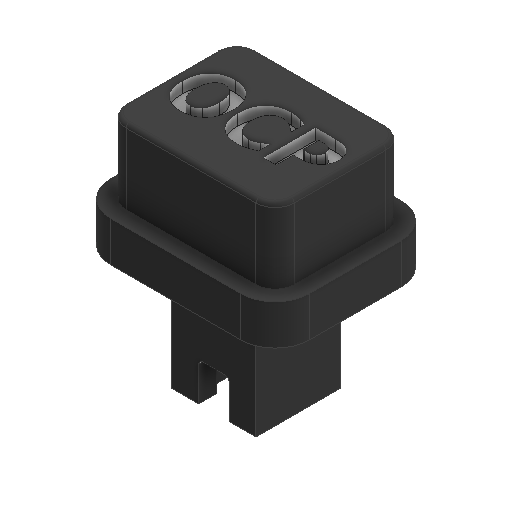
# Autodesk Inventor part: Button cap
Saved by Autodesk Inventor 2025 (Build 290162000, 162)
## iProperties
Created: 2025-01-02
Part Number: Button cap
Material: Generic
Document SubType Name: Modeling
Designer: Jan Mareš
Density: 1 g/cm^3
Appearance: Default
Author: Jan Mareš
Autodesk Inventor part; units mm, degrees
ref_plane "YZ Plane" through (0, 0, 0) normal (1, 0, 0) x (0, 1, 0)
ref_plane "XZ Plane" through (0, 0, 0) normal (0, 1, 0) x (-1, 0, 0)
ref_plane "XY Plane" through (0, 0, 0) normal (0, 0, 1) x (1, 0, 0)
sketch "Sketch1" plane through (0, 0, 0) normal (0, 1, 0) x (-1, 0, 0)
  line L0 (3.08, 0) -> (-3.08, 0) construction
  line L1 (0, -3.08) -> (0, 3.08) construction
  line L2 (-2.2, 2.2) -> (2.2, 2.2)
  line L3 (2.2, 2.2) -> (2.2, -2.2)
  line L4 (2.2, -2.2) -> (-2.2, -2.2)
  line L5 (-2.2, -2.2) -> (-2.2, 2.2)
  line L6 (-2.2, 0) -> (2.2, 0) construction
  point P0 (0, 0)
  dimension "d0" = 4.4
  constraints: 10 end point, 3 midpoint, 2 parallel, 2 perpendicular, 1 horizontal
  measures "d0" distance of L2.start L2.end
extrude "Extrusion1" add sketch "Sketch1" along normal blind 6
sketch "Sketch2" plane through (0, 0, 0) normal (0, -1, 0) x (1, 0, 0)
  line L0 (-1.25, 1.25) -> (1.25, 1.25)
  line L1 (1.25, 1.25) -> (1.25, -1.25)
  line L2 (1.25, -1.25) -> (-1.25, -1.25)
  line L3 (-1.25, -1.25) -> (-1.25, 1.25)
  line L4 (-1.25, 0) -> (1.25, 0) construction
  point P0 (0, 0)
  point P1 (0, 0)
  dimension "d3" = 2.5
  constraints: 10 end point, 3 midpoint, 2 parallel, 2 perpendicular, 1 coincident, 1 horizontal
  measures "d3" distance of L0.start L0.end
extrude "Extrusion2" cut sketch "Sketch2" against normal blind 2.8
sketch "Sketch3" plane through (-2.2, 0, 2.2) normal (0, 0, 1) x (1, 0, 0)
  line L0 (2.2, -1.2) -> (2.2, 7.2) construction
  line L1 (-0.88, 0) -> (5.28, 0) construction
  line L2 (1.4, 0) -> (1.4, 2)
  line L3 (1.4, 2) -> (3, 2)
  line L4 (3, 2) -> (3, 0)
  line L5 (1.4, 0) -> (3, 0)
  line L6 (1.4, 1) -> (3, 1) construction
  point P0 (2.2, 0)
  point P1 (2.2, 1)
  dimension "d6" = 1.6
  dimension "d7" = 2
  constraints: 10 end point, 3 midpoint, 3 point on line, 2 perpendicular, 1 collinear, 1 vertical
  measures "d6" distance of L2.end L3.end
  measures "d7" distance of L3.end L4.end
extrude "Extrusion3" cut sketch "Sketch3" against normal through all
sketch "Sketch4" plane through (0, 0, 0) normal (0, 0, 1) x (1, 0, 0)
  line L0 (1.25, 0) -> (1.25, 2.8) construction
  line L1 (-1.25, 0) -> (-1.25, 2.8) construction
  line L2 (-1.758, 0) -> (1.798, 0) construction
  arc A0 (1.25, 0.9) -> (1.25, 0.6317) centre (1.29, 0.7658) ccw
  line L3 (1.29, 0.7658) -> (1.15, 0.7658) construction
  line L4 (1.25, 0.6317) -> (1.25, 0.9) construction
  line L5 (1.1441, 0.9) -> (1.25, 0.9)
  line L6 (1.1441, 0.9) -> (1.25, 0.7165)
  line L7 (1.25, 0.9) -> (1.25, 0.7165)
  line L8 (1.25, 0.9) -> (1.25, 0.6317)
  point P0 (0, 0)
  dimension "d13" = 0.1
  dimension "d14" = 1.9
  dimension "d15" = 0.14
  dimension "d28" = 30
  dimension "d29" = 0.106
  dimension "d30" = 1.9
  constraints: 12 end point, 6 point on line, 3 point on circle, 1 centre point, 1 collinear, 1 horizontal, 1 perpendicular
  measures "d13" distance from line of L0 L3.end
  measures "d14" distance of L4.end L0.end
  measures "d15" radius of A0
  measures "d28" angle of L0 L6
  measures "d29" distance of L5.start L5.end
  measures "d30" distance from line of L5 L0.end
extrude "Extrusion4" add sketch "Sketch4" along normal through all both and the other way through all contours L7 L6 A0 | L6 L8 A0
mirror "Mirror1" about plane through (0, 0, 0) normal (1, 0, 0) of "Extrusion4"
sketch "Sketch5" plane through (0, 6, 0) normal (0, 1, 0) x (1, 0, 0)
  line L0 (-4.4, -3.4) -> (4.4, -3.4)
  line L1 (4.4, -3.4) -> (4.4, 3.4)
  line L2 (4.4, 3.4) -> (-4.4, 3.4)
  line L3 (-4.4, 3.4) -> (-4.4, -3.4)
  line L4 (0, -3.4) -> (0, 3.4) construction
  line L5 (6.16, 0) -> (-6.16, 0) construction
  point P0 (0, 0)
  dimension "d18" = 6.8
  dimension "d19" = 8.8
  constraints: 10 end point, 3 midpoint, 2 parallel, 1 horizontal, 1 perpendicular
  measures "d18" distance of L2.end L0.start
  measures "d19" distance of L0.start L0.end
extrude "Extrusion5" add sketch "Sketch5" along normal blind 6
fillet "Fillet1" radius 1 4 edges at (4.4, 9, 3.4) (4.4, 9, -3.4) (-4.4, 9, 3.4) (-4.4, 9, -3.4)
fillet "Fillet2" radius 0.2 8 edges at (4.1071, 12, -3.1071) (0, 12, -3.4) (-4.1071, 12, -3.1071) (-4.4, 12, 0) (-4.1071, 12, 3.1071) (0, 12, 3.4) (4.1071, 12, 3.1071) (4.4, 12, 0)
sketch "Sketch6" plane through (0, 6, 0) normal (0, -1, 0) x (1, 0, 0)
  line L0 (-3.4, 3.4) -> (3.4, 3.4) projected
  arc A0 (4.4, 2.4) -> (3.4, 3.4) centre (3.4, 2.4) ccw projected
  line L1 (4.4, 2.4) -> (4.4, -2.4) projected
  arc A1 (3.4, -3.4) -> (4.4, -2.4) centre (3.4, -2.4) ccw projected
  line L2 (3.4, -3.4) -> (-3.4, -3.4) projected
  arc A2 (-4.4, -2.4) -> (-3.4, -3.4) centre (-3.4, -2.4) ccw projected
  line L3 (-4.4, -2.4) -> (-4.4, 2.4) projected
  arc A3 (-3.4, 3.4) -> (-4.4, 2.4) centre (-3.4, 2.4) ccw projected
  line L4 (3.4, 4.2) -> (-3.4, 4.2)
  arc A4 (-3.4, 4.2) -> (-5.2, 2.4) centre (-3.4, 2.4) ccw
  line L5 (-5.2, 2.4) -> (-5.2, -2.4)
  arc A5 (-5.2, -2.4) -> (-3.4, -4.2) centre (-3.4, -2.4) ccw
  line L6 (-3.4, -4.2) -> (3.4, -4.2)
  arc A6 (3.4, -4.2) -> (5.2, -2.4) centre (3.4, -2.4) ccw
  line L7 (5.2, -2.4) -> (5.2, 2.4)
  arc A7 (5.2, 2.4) -> (3.4, 4.2) centre (3.4, 2.4) ccw
  point P0 (0, 0)
  dimension "d24" = 0.8
  constraints: 8 end point, 8 point on circle, 4 centre point, 7 other
  measures "d24" distance between parallel lines of L0 L4
extrude "Extrusion6" add sketch "Sketch6" against normal blind 2.1
fillet "Fillet3" radius 0.6 4 edges at (0, 6, 2.2) (-2.2, 6, 0) (2.2, 6, 0) (0, 6, -2.2)
fillet "Fillet4" radius 0.2 4 edges at (0, 2.8, 1.25) (-1.25, 2.8, 0) (0, 2.8, -1.25) (1.25, 2.8, 0)
fillet "Fillet5" radius 0.2 4 edges at (0.8, 2, 1.725) (-0.8, 2, 1.725) (-0.8, 2, -1.725) (0.8, 2, -1.725)
sketch "Sketch7" plane through (0, 12, 0) normal (0, 1, 0) x (1, 0, 0)
  line L0 (-4, 1.45) -> (3.9, 1.45) construction
  line L1 (3.9, 1.45) -> (3.9, -1.7675) construction
  line L2 (3.9, -1.7675) -> (-4, -1.7675) construction
  line L3 (-4, -1.7675) -> (-4, 1.45) construction
  line L4 (-4.4, 2.4) -> (-4.4, -2.4) projected
  line L5 (4.4, -2.4) -> (4.4, 2.4) projected
  line L6 (-2.5439, -1.3268) -> (-2.5439, -3.4)
  line L7 (-3.4, -3.4) -> (3.4, -3.4) projected
  line L8 (-2.5439, 1.45) -> (-2.5439, 3.3876)
  line L9 (3.4, 3.4) -> (-3.4, 3.4) projected
  line L10 (-2.119, 1.5763) -> (-2.119, 3.4)
  spline S0 degree 2 poles (-1.2121, 0.0171) (-1.2121, -0.6515) (-1.9252, -1.4159) (-2.5448, -1.4159) knots 0 0 0 1 2 2 2
  spline S1 degree 2 poles (-2.5448, -1.4159) (-3.1665, -1.4159) (-3.8752, -0.6426) (-3.8752, 0.0171) knots 0 0 0 1 2 2 2
  spline S2 degree 2 poles (-3.8752, 0.0171) (-3.8752, 0.6789) (-3.1665, 1.45) (-2.5448, 1.45) knots 0 0 0 1 2 2 2
  spline S3 degree 2 poles (-2.5448, 1.45) (-1.9252, 1.45) (-1.2121, 0.6834) (-1.2121, 0.0171) knots 0 0 0 1 2 2 2
  spline S4 degree 2 poles (-1.9252, 0.0171) (-1.9252, 0.2644) (-2.0255, 0.6098) (-2.1124, 0.719) knots 0 0 0 1 2 2 2
  spline S5 degree 2 poles (-2.1124, 0.719) (-2.1994, 0.8327) (-2.4222, 0.9308) (-2.5425, 0.9308) knots 0 0 0 1 2 2 2
  spline S6 degree 2 poles (-2.5425, 0.9308) (-2.6696, 0.9308) (-2.8768, 0.8394) (-2.9726, 0.7235) knots 0 0 0 1 2 2 2
  spline S7 degree 2 poles (-2.9726, 0.7235) (-3.0573, 0.6165) (-3.1621, 0.2622) (-3.1621, 0.0171) knots 0 0 0 1 2 2 2
  spline S8 degree 2 poles (-3.1621, 0.0171) (-3.1621, -0.237) (-3.0618, -0.5713) (-2.9749, -0.6849) knots 0 0 0 1 2 2 2
  spline S9 degree 2 poles (-2.9749, -0.6849) (-2.888, -0.7986) (-2.6629, -0.8966) (-2.5425, -0.8966) knots 0 0 0 1 2 2 2
  spline S10 degree 2 poles (-2.5425, -0.8966) (-2.42, -0.8966) (-2.1927, -0.7919) (-2.1102, -0.6805) knots 0 0 0 1 2 2 2
  spline S11 degree 2 poles (-2.1102, -0.6805) (-2.0211, -0.5601) (-1.9252, -0.2415) (-1.9252, 0.0171) knots 0 0 0 1 2 2 2
  spline S12 degree 2 poles (0.3835, -1.4114) (-0.236, -1.4114) (-0.9625, -0.6626) (-0.9625, 0.0148) knots 0 0 0 1 2 2 2
  spline S13 degree 2 poles (-0.9625, 0.0148) (-0.9625, 0.6678) (-0.2338, 1.4455) (0.3857, 1.4455) knots 0 0 0 1 2 2 2
  spline S14 degree 2 poles (0.3857, 1.4455) (0.5484, 1.4455) (0.8114, 1.4077) (0.9317, 1.3765) knots 0 0 0 1 2 2 2
  spline S15 degree 2 poles (0.9317, 1.3765) (1.0253, 1.3475) (1.2459, 1.2517) (1.315, 1.216) knots 0 0 0 1 2 2 2
  line L11 (1.315, 1.216) -> (1.315, 0.5608)
  line L12 (1.315, 0.5608) -> (1.2459, 0.5608)
  spline S16 degree 2 poles (1.2459, 0.5608) (1.1947, 0.6054) (1.0432, 0.7302) (0.9473, 0.7881) knots 0 0 0 1 2 2 2
  spline S17 degree 2 poles (0.9473, 0.7881) (0.8515, 0.8483) (0.622, 0.9308) (0.4949, 0.9308) knots 0 0 0 1 2 2 2
  spline S18 degree 2 poles (0.4949, 0.9308) (0.3456, 0.9308) (0.0983, 0.8372) (-0.0154, 0.719) knots 0 0 0 1 2 2 2
  spline S19 degree 2 poles (-0.0154, 0.719) (-0.1179, 0.6143) (-0.2494, 0.2555) (-0.2494, 0.0126) knots 0 0 0 1 2 2 2
  spline S20 degree 2 poles (-0.2494, 0.0126) (-0.2494, -0.2437) (-0.1135, -0.5936) (-0.002, -0.7005) knots 0 0 0 1 2 2 2
  spline S21 degree 2 poles (-0.002, -0.7005) (0.1049, -0.8053) (0.3679, -0.8966) (0.4994, -0.8966) knots 0 0 0 1 2 2 2
  spline S22 degree 2 poles (0.4994, -0.8966) (0.6353, -0.8966) (0.8827, -0.8053) (0.9674, -0.7496) knots 0 0 0 1 2 2 2
  spline S23 degree 2 poles (0.9674, -0.7496) (1.061, -0.6938) (1.2014, -0.5757) (1.2526, -0.5289) knots 0 0 0 1 2 2 2
  line L13 (1.2526, -0.5289) -> (1.315, -0.5289)
  line L14 (1.315, -0.5289) -> (1.315, -1.1752)
  spline S24 degree 2 poles (1.315, -1.1752) (1.2393, -1.2109) (1.0409, -1.3) (0.934, -1.3312) knots 0 0 0 1 2 2 2
  spline S25 degree 2 poles (0.934, -1.3312) (0.8047, -1.3713) (0.5796, -1.4114) (0.3835, -1.4114) knots 0 0 0 1 2 2 2
  spline S26 degree 2 poles (3.8377, 0.5252) (3.8377, 0.3335) (3.7152, -0.0141) (3.6015, -0.13) knots 0 0 0 1 2 2 2
  spline S27 degree 2 poles (3.6015, -0.13) (3.5324, -0.2036) (3.363, -0.3239) (3.2628, -0.3662) knots 0 0 0 1 2 2 2
  spline S28 degree 2 poles (3.2628, -0.3662) (3.1603, -0.4086) (2.9218, -0.4576) (2.7747, -0.4576) knots 0 0 0 1 2 2 2
  line L15 (2.7747, -0.4576) -> (2.4137, -0.4576)
  line L16 (2.4137, -0.4576) -> (2.4137, -1.3579)
  line L17 (2.4137, -1.3579) -> (1.7229, -1.3579)
  line L18 (1.7229, -1.3579) -> (1.7229, 1.3921)
  line L19 (1.7229, 1.3921) -> (2.7903, 1.3921)
  spline S29 degree 2 poles (2.7903, 1.3921) (3.0265, 1.3921) (3.372, 1.3051) (3.5124, 1.2115) knots 0 0 0 1 2 2 2
  spline S30 degree 2 poles (3.5124, 1.2115) (3.6684, 1.1068) (3.8377, 0.7636) (3.8377, 0.5252) knots 0 0 0 1 2 2 2
  spline S31 degree 2 poles (3.1291, 0.5073) (3.1291, 0.6254) (3.0176, 0.7926) (2.9419, 0.8238) knots 0 0 0 1 2 2 2
  spline S32 degree 2 poles (2.9419, 0.8238) (2.8438, 0.8661) (2.6655, 0.8795) (2.5118, 0.8795) knots 0 0 0 1 2 2 2
  line L20 (2.5118, 0.8795) -> (2.4137, 0.8795)
  line L21 (2.4137, 0.8795) -> (2.4137, 0.0549)
  line L22 (2.4137, 0.0549) -> (2.4627, 0.0549)
  spline S33 degree 2 poles (2.4627, 0.0549) (2.5585, 0.0549) (2.7324, 0.0594) (2.797, 0.0705) knots 0 0 0 1 2 2 2
  spline S34 degree 2 poles (2.797, 0.0705) (2.8527, 0.0795) (2.9753, 0.1329) (3.0087, 0.1664) knots 0 0 0 1 2 2 2
  spline S35 degree 2 poles (3.0087, 0.1664) (3.08, 0.2332) (3.1291, 0.3825) (3.1291, 0.5073) knots 0 0 0 1 2 2 2
  point P0 (0, 0)
  dimension "d33" = 0.4
  dimension "d34" = 0.5
  dimension "d37" = 1.95
  constraints: 6 end point, 5 point on line, 1 perpendicular, 1 vertical, 2 other
  measures "d33" distance between parallel lines of L3 L4
  measures "d34" distance between parallel lines of L5 L1
  measures "d37" distance between parallel lines of L0 L9
emboss "Emboss1" sketch "Sketch7" operation cut depth 0.6 direction (0, -1, 0)
ref_plane "Work Plane1" through (0, 0, 0) normal (1, 0, 0) x (0, 1, 0)
body "Solid1"
